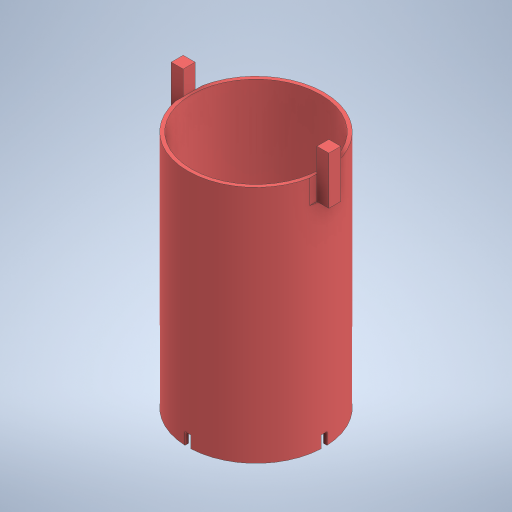
# Autodesk Inventor part: Cooking Pipe
Saved by Autodesk Inventor 2024.3 (Build 283343000, 343)
## iProperties
Created: 2025-03-01
Part Number: Cooking Pipe
Material: Generic
Document SubType Name: Modeling
Designer: ajclo
Density: 1 g/cm^3
Appearance: Default
Author: ajclo
Autodesk Inventor part; units mm, degrees
ref_plane "YZ Plane" through (0, 0, 0) normal (1, 0, 0) x (0, 1, 0)
ref_plane "XZ Plane" through (0, 0, 0) normal (0, 1, 0) x (-1, 0, 0)
ref_plane "XY Plane" through (0, 0, 0) normal (0, 0, 1) x (1, 0, 0)
sketch "Sketch1" plane through (0, 0, 0) normal (0, 1, 0) x (-1, 0, 0)
  circle A0 centre (0, 0) radius 54
  circle A1 centre (0, 0) radius 57
  dimension "d0" = 3
  dimension "d1" = 114
  constraints: 2 centre point, 2 coincident
  measures "d0" radial gap between concentric circles of A1 A0
  measures "d1" diameter of A1
extrude "Extrusion1" add sketch "Sketch1" along normal blind 200
sketch "Sketch2" plane through (0, 200, 0) normal (0, 1, 0) x (1, 0, 0)
  circle A0 centre (0, 0) radius 57 projected
  line L0 (55.9285, -11) -> (-55.9285, -11)
  line L1 (-55.9285, -11) -> (-55.9285, 11)
  line L2 (-55.9285, 11) -> (55.9285, 11)
  line L3 (55.9285, 11) -> (55.9285, -11)
  line L4 (55.9285, -11) -> (-55.9285, 11) construction
  line L5 (-55.9285, -11) -> (55.9285, 11) construction
  dimension "d4" = 22
  constraints: 12 end point, 2 midpoint, 2 parallel, 1 horizontal, 1 perpendicular, 1 point on circle
  measures "d4" distance of L0.end L1.end
extrude "Extrusion2" cut sketch "Sketch2" against normal blind 20 contours A0 L3 | L1 A0
sketch "Sketch3" plane through (-55.9285, 200, -11) normal (-1, 0, 0) x (0, 0, 1)
  line L0 (0, -20) -> (22, -20) projected
  line L1 (16, -20) -> (6, -20)
  line L2 (6, -20) -> (6, 20)
  line L3 (6, 20) -> (16, 20)
  line L4 (16, 20) -> (16, -20)
  line L5 (0, -20) -> (0, 0) projected
  point P0 (11, -200)
  point P1 (6, 0)
  point P2 (6, -20)
  dimension "d7" = 40
  dimension "d8" = 10
  dimension "d9" = 6
  constraints: 8 end point, 2 parallel, 1 horizontal, 1 midpoint, 1 perpendicular, 1 point on line
  measures "d7" distance of L3.end L1.start
  measures "d8" distance of L2.end L3.end
  measures "d9" distance from line of L5 point (6, 0)
extrude "Extrusion3" add sketch "Sketch3" along normal blind 10
mirror "Mirror1" about plane through (0, 0, 0) normal (1, 0, 0) of "Extrusion3"
sketch "Sketch4" plane through (0, 0, 0) normal (0, -1, 0) x (1, 0, 0)
  line L0 (-2.5, -60) -> (2.5, -60)
  line L1 (2.5, -60) -> (2.5, 60)
  line L2 (2.5, 60) -> (-2.5, 60)
  line L3 (-2.5, 60) -> (-2.5, -60)
  line L4 (-2.5, -60) -> (2.5, 60) construction
  line L5 (2.5, -60) -> (-2.5, 60) construction
  line L6 (60, -2.5) -> (-60, -2.5)
  line L7 (-60, -2.5) -> (-60, 2.5)
  line L8 (-60, 2.5) -> (60, 2.5)
  line L9 (60, 2.5) -> (60, -2.5)
  line L10 (60, -2.5) -> (-60, 2.5) construction
  line L11 (-60, -2.5) -> (60, 2.5) construction
  point P0 (0, 0)
  point P1 (-2.5, -2.5)
  point P2 (2.5, -2.5)
  point P3 (2.5, 2.5)
  point P4 (-2.5, 2.5)
  dimension "d12" = 5
  dimension "d13" = 5
  dimension "d14" = 120
  dimension "d15" = 120
  constraints: 24 end point, 4 midpoint, 4 parallel, 2 horizontal, 2 perpendicular
  measures "d12" distance of L1.end L2.end
  measures "d13" distance of L6.end L7.end
  measures "d14" distance of L2.end L0.start
  measures "d15" distance of L7.end L8.end
extrude "Extrusion4" cut sketch "Sketch4" against normal blind 10
equation "\"d13\" = d12"
equation "\"d15\" = d14"
body "Solid1"
